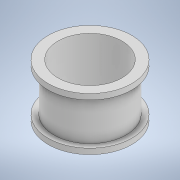
# Autodesk Inventor part: inner tube
Saved by Autodesk Inventor 2021 (Build 250183000, 183)
## iProperties
Created: 2022-11-02
Part Number: inner tube
Material: Generic
Document SubType Name: Modeling
Designer: warre
Density: 1 g/cm^3
Appearance: Default
Author: warre
Autodesk Inventor part; units mm, degrees
ref_plane "YZ Plane" through (0, 0, 0) normal (1, 0, 0) x (0, 1, 0)
ref_plane "XZ Plane" through (0, 0, 0) normal (0, 1, 0) x (-1, 0, 0)
sketch "Sketch1" plane through (0, 0, 0) normal (0, 1, 0) x (-1, 0, 0)
  circle A0 centre (0, 0) radius 13
  circle A1 centre (0, 0) radius 11.5
  dimension "d0" = 26
  dimension "d1" = 23
  constraints: 2 centre point, 2 coincident
  measures "d0" diameter of A0
  measures "d1" diameter of A1
extrude "Extrusion1" add sketch "Sketch1" along normal blind 15
sketch "Sketch2" plane through (0, 15, 0) normal (0, 1, 0) x (1, 0, 0)
  circle A0 centre (0, 0) radius 15
  circle A1 centre (0, 0) radius 11.5 projected
  dimension "d4" = 30
  constraints: 1 centre point, 1 coincident
  measures "d4" diameter of A0
extrude "Extrusion2" add sketch "Sketch2" along normal blind 2
ref_plane "Work Plane1" through (0, 7.5, 0) normal (0, -1, 0) x (1, 0, 0)
mirror "Mirror1" about plane through (0, 7.5, 0) normal (0, -1, 0) of "Extrusion2"
body "Solid1"
